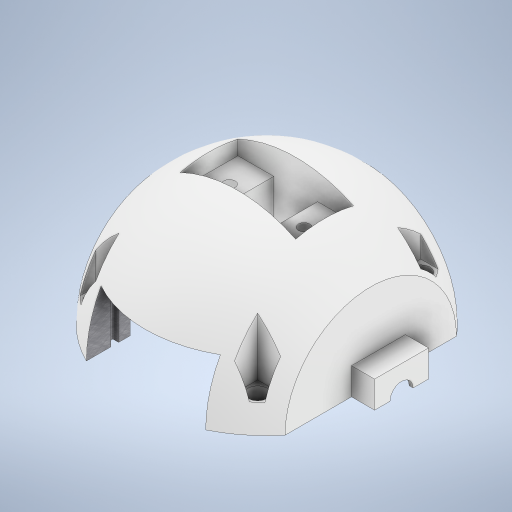
# Autodesk Inventor part: naibu-rightside
Saved by Autodesk Inventor 2023 (Build 270158000, 158)
## iProperties
Created: 2022-10-08
Part Number: naibu-rightside
Material: ABS プラスチック
Document SubType Name: Modeling
Designer: ellie
Density: 1.06 g/cm^3
Appearance: 積雪
Author: ellie
Autodesk Inventor part; units mm, degrees
ref_plane "YZ Plane" through (0, 0, 0) normal (1, 0, 0) x (0, 1, 0)
ref_plane "XZ Plane" through (0, 0, 0) normal (0, 1, 0) x (-1, 0, 0)
ref_plane "XY Plane" through (0, 0, 0) normal (0, 0, 1) x (1, 0, 0)
sketch "スケッチ1" plane through (0, 0, 0) normal (0, 1, 0) x (-1, 0, 0)
  circle A0 centre (0, 0) radius 35
  line L0 (0, 0) -> (0, -35)
  line L1 (0, 0) -> (0, 35)
  dimension "d0" = 70
  constraints: 4 end point, 2 point on circle, 2 vertical, 1 centre point, 1 coincident
  measures "d0" diameter of A0
revolve "回転1" add sketch "スケッチ1" angle 180 about axis through (0, 0, 0) along (0, 0, 1) picked at (-2.5961, -23.0408) contours L1 L0 A0
sketch "スケッチ5" plane through (0, 0, 0) normal (0, -1, 0) x (1, 0, 0)
  line L0 (-20, -23) -> (20, -23)
  line L1 (20, -23) -> (20, -13)
  line L2 (20, -13) -> (-20, -13)
  line L3 (-20, -13) -> (-20, -23)
  line L4 (-20, -15) -> (-20, -13)
  line L5 (0, 25) -> (-17, 25)
  line L6 (-17, 25) -> (-17, 23)
  line L7 (-17, 23) -> (0, 23)
  line L8 (0, 23) -> (0, 25)
  line L9 (0, 20) -> (-20, 20)
  line L10 (-20, 20) -> (-20, 19)
  line L11 (-20, 19) -> (0, 19)
  line L12 (0, 19) -> (0, 20)
  line L13 (0, 13) -> (-21, 13)
  line L14 (-21, 13) -> (-21, 11)
  line L15 (-21, 11) -> (0, 11)
  line L16 (0, 11) -> (0, 13)
  line L17 (0, 5) -> (-23, 5)
  line L18 (-23, 5) -> (-23, 3)
  line L19 (-23, 3) -> (0, 3)
  line L20 (0, 3) -> (0, 5)
  circle A0 centre (0, 0) radius 35 projected
  circle A1 centre (0, 0) radius 35 projected
  line L21 (0, 35) -> (0, -35)
  line L22 (35, 0) -> (-35, 0)
  line L23 (-32, 3) -> (-23, 3)
  line L24 (-23, 3) -> (-23, -7)
  line L25 (-23, -7) -> (-32, -7)
  line L26 (-32, -7) -> (-32, 3)
  line L27 (-23, -8.0262) -> (-23, 3)
  line L28 (-27, 22.2711) -> (-27, -22.2711)
  line L29 (-15.5, 25) -> (0, 25)
  line L30 (0, 25) -> (0, 35)
  line L31 (0, 35) -> (-15.5, 35)
  line L32 (-15.5, 35) -> (-15.5, 25)
  line L33 (-15.5, 23) -> (0, 23)
  line L34 (0, 23) -> (0, 20)
  line L35 (0, 20) -> (-15.5, 20)
  line L36 (-15.5, 20) -> (-15.5, 23)
  line L37 (-19, 13) -> (0, 13)
  line L38 (0, 13) -> (0, 19)
  line L39 (0, 19) -> (-19, 19)
  line L40 (-19, 19) -> (-19, 13)
  line L41 (-19, 11) -> (0, 11)
  line L42 (0, 11) -> (0, 5)
  line L43 (0, 5) -> (-19, 5)
  line L44 (-19, 5) -> (-19, 11)
  line L45 (-23, -2) -> (-39.6865, -2)
  line L46 (-23, -2) -> (-7.8337, -2)
  line L47 (-8, 3) -> (-23, 3)
  line L48 (-23, 3) -> (-23, -7)
  line L49 (-23, -7) -> (-8, -7)
  line L50 (-8, -7) -> (-8, 3)
  line L51 (-8, 3) -> (-23, -7) construction
  line L52 (-23, 3) -> (-8, -7) construction
  line L53 (-23, 5) -> (-33, 5)
  line L54 (-33, 5) -> (-33, -9)
  line L55 (-33, -9) -> (-23, -9)
  line L56 (-23, -9) -> (-23, 5)
  line L57 (-23, 5) -> (-33, -9) construction
  line L58 (-33, 5) -> (-23, -9) construction
  line L59 (-8, 3) -> (-1, 3)
  line L60 (-1, 3) -> (-1, -7)
  line L61 (-1, -7) -> (-8, -7)
  line L62 (-8, -7) -> (-8, 3)
  line L63 (-8, 3) -> (-1, -7) construction
  line L64 (-1, 3) -> (-8, -7) construction
  line L65 (-23, 3) -> (-27, 3)
  line L66 (-23, -7) -> (-27, -7)
  line L67 (-23, 5) -> (-27, 5)
  line L68 (-23, -9) -> (-27, -9)
  line L69 (23.4307, -26) -> (-23.4307, -26)
  line L70 (-8, 3) -> (-6.8, 3)
  line L71 (-6.8, 3) -> (-6.8, -7)
  line L72 (-6.8, -7) -> (-8, -7)
  line L73 (-8, -7) -> (-8, 3)
  line L74 (0, 5) -> (2, 5)
  line L75 (0, -3) -> (0, 5)
  line L76 (-11.5791, -13) -> (-8, -13)
  point P0 (0, -23)
  point P1 (0, -13)
  point P2 (0, 24)
  point P3 (0, 19.5)
  point P4 (0, 12)
  point P5 (0, 4)
  point P6 (-20, -18)
  point P7 (-27, -0.5262)
  point P8 (-27, -7)
  point P9 (-15.5, 21.5)
  point P10 (-15.5, 31.3807)
  point P11 (0, 25)
  point P12 (0, 23)
  point P13 (0, 11)
  point P14 (0, 13)
  point P15 (-27, 0)
  point P16 (-32, 0)
  point P17 (-23, 0)
  point P18 (-15.5, -2)
  point P19 (-28, -2)
  point P20 (-4.5, -2)
  point P21 (-8, -7)
  point P22 (-8, 3)
  point P23 (-27, 0.5)
  point P24 (-28, 0.4738)
  point P25 (-28, -11.5262)
  point P26 (-27, -11.5)
  point P27 (-23, 3)
  point P28 (-8, 0)
  point P29 (-1, 0)
  point P30 (-8, -7)
  point P31 (0, 5)
  point P32 (0, 3)
  point P33 (-27, -9)
  point P34 (-27, 5)
  dimension "d12" = 40
  dimension "d13" = 10
  dimension "d23" = 17
  dimension "d24" = 2
  dimension "d27" = 20
  dimension "d28" = 1
  dimension "d30" = 21
  dimension "d31" = 2
  dimension "d33" = 2
  dimension "d88" = 0
  dimension "d89" = 0
  dimension "d90" = 12
  dimension "d92" = 20
  dimension "d93" = 10
  dimension "d97" = 9
  dimension "d98" = 10
  dimension "d113" = 27
  dimension "d122" = 15.5
  dimension "d123" = 35
  dimension "d124" = 3
  dimension "d125" = 15.5
  dimension "d126" = 6
  dimension "d127" = 6
  dimension "d147" = 10
  dimension "d149" = 8
  dimension "d151" = 15
  dimension "d161" = 14
  dimension "d162" = 10
  dimension "d164" = 10
  dimension "d165" = 7
  dimension "d170" = 26
  dimension "d175" = 1.2
  dimension "d187" = 1
  dimension "d262" = 2
  dimension "d263" = 2
  constraints: 152 end point, 29 parallel, 19 horizontal, 17 perpendicular, 15 midpoint, 15 point on line, 9 collinear, 1 vertical, 20 other
  measures "d12" distance of L2.end L1.end
  measures "d13" distance of L1.end L0.end
  measures "d23" distance of L7.end L6.end
  measures "d24" distance of L6.end L5.end
  measures "d27" distance of L11.end L10.end
  measures "d28" distance of L10.end L9.end
  measures "d30" distance of L15.end L14.end
  measures "d31" distance of L14.end L13.end
  measures "d33" distance of L18.end L17.end
  measures "d89" distance from line of point (0, 0) L22
  measures "d90" distance from line of L0 point (0, -35)
  measures "d92" distance of the line from the sketch origin of L3
  measures "d93" distance from line of L5 point (0, 35)
  measures "d97" distance of L24.end L25.end
  measures "d98" distance of L23.end L24.end
  measures "d113" distance of the line from the sketch origin of L28
  measures "d122" distance of the line from the sketch origin of L32
  measures "d123" distance between parallel lines of L31 L22
  measures "d124" distance of L33.end L34.end
  measures "d126" distance of L38.end L37.end
  measures "d127" distance of L41.end L42.end
  measures "d147" distance of L48.end L47.end
  measures "d149" distance of the line from the sketch origin of L50
  measures "d151" distance between parallel lines of L50 L24
  measures "d161" distance between parallel lines of L55 L53
  measures "d162" distance between parallel lines of L48 L54
  measures "d164" distance between parallel lines of L61 L59
  measures "d165" distance between parallel lines of L50 L60
  measures "d170" distance between parallel lines of L69 L22
  measures "d175" distance of L71.end L72.end
  measures "d187" distance between parallel lines of L75 L60
  measures "d262" distance between parallel lines of L14 L44
  measures "d263" distance between parallel lines of L14 L40
extrude "GNSボード" cut sketch "スケッチ5" against normal blind 16 contours L8 L7 L6 L5
extrude "GNSボード止めるよう" cut sketch "スケッチ5" against normal blind 15 contours L21 L5 L32 A0 | L21 L9 L36 L7
extrude "アルミ板１" cut sketch "スケッチ5" against normal blind 20 contours L12 L11 L10 L9
extrude "メイン基板" cut sketch "スケッチ5" against normal blind 21 contours L15 L14 L13 L16
extrude "メイン止めるよう" cut sketch "スケッチ5" against normal blind 16.5 contours L17 L44 L15 L21 | L13 L40 L11 L21
extrude "アルミ板２" cut sketch "スケッチ5" against normal blind 20 contours L19 L18 L17 L20
extrude "電池ボックス入れ" cut sketch "スケッチ5" against normal blind 13 contours L3 L2 L21 L0 | L21 L2 L1 L0
extrude "side ut" cut sketch "スケッチ5" against normal blind 100 contours A0 L45 L54 L55 L28 | A0 L22 L54 L45 | L55 L54 L45 L26 L25 L28 | A0 L28 L53 L54 L22 | L54 L22 L26 L45 | L25 L26 L45 L28 | L54 L53 L28 L23 L26 L22 | L26 L22 L28 L45 | L26 L23 L28 L22
extrude "motor case" add sketch "スケッチ5" against normal blind 7 contours L55 L54 L45 L26 L25 L28 | L28 L25 L27 L56 L55 | L54 L22 L26 L45 | L28 L45 L24 L25 | L25 L26 L45 L28 | L50 L46 L24 L22 | L22 L24 L19 L50 | L54 L53 L28 L23 L26 L22 | L26 L22 L28 L45 | L24 L46 L50 L49 | L28 L22 L24 L45 | L18 L23 L28 L53 | L22 L28 L23 L24 | L26 L23 L28 L22
extrude "bottom cut" cut sketch "スケッチ5" against normal blind 90 contours L69 A0 L21 | L21 A0 L69
extrude "motor" cut sketch "スケッチ5" against normal blind 6 contours L60 L61 L71 L22 | L22 L71 L19 L60 | L71 L61 L50 L22 | L22 L50 L19 L71 | L28 L45 L24 L25 | L25 L26 L45 L28 | L50 L46 L24 L22 | L22 L24 L19 L50 | L26 L22 L28 L45 | L24 L46 L50 L49 | L28 L22 L24 L45 | L22 L28 L23 L24 | L26 L23 L28 L22
extrude "motor block" add sketch "スケッチ5" against normal blind 10 contours L71 L61 L50 L22 | L22 L50 L19 L71
sketch "スケッチ26" plane through (-33, 0, -9) normal (-1, 0, 0) x (0, 0, 1)
  line L0 (14, 0) -> (0, 0) projected
  circle A0 centre (7, 0) radius 3
  point P0 (9, 0)
  point P1 (7, 0)
  point P2 (7, 0)
  point P3 (7, 0)
  point P4 (4, 0)
  point P5 (10, 0)
  dimension "d197" = 6
  constraints: 1 centre point, 1 coincident
  measures "d197" diameter of A0
extrude "押し出し34" cut sketch "スケッチ26" against normal blind 27 contours L0 A0 picked at (7.7485, 0.6631)
mirror "ミラー11" about plane through (0, 0, 0) normal (1, 0, 0) of "GNSボード", "GNSボード止めるよう", "アルミ板１", "メイン止めるよう", "メイン基板", "アルミ板２", "motor", "押し出し34", "motor case", "電池ボックス入れ", "motor block", "side ut"
ref_plane "作業平面5" through (0, 13, 0) normal (0, -1, 0) x (1, 0, 0)
ref_plane "作業平面6" through (-15.5, 35, 25) normal (0, -1, 0) x (1, 0, 0)
sketch "スケッチ29" plane through (-15.5, 35, 25) normal (0, -1, 0) x (1, 0, 0)
  line L0 (15.5, -25) -> (-67.7134, -25)
  line L1 (-67.7134, -25) -> (15.5, -25)
  line L2 (110.7852, -24.5555) -> (110.7852, -27.3413)
  line L3 (15.5, -25) -> (98.1975, -25)
  circle A0 centre (25.2, -25) radius 1.5
  circle A1 centre (5.8, -25) radius 1.5
  line L4 (32.5, 0) -> (-1.5, 0) projected
  line L5 (15.5, 0) -> (15.5, -51)
  line L6 (-7.9307, -51) -> (38.9307, -51) projected
  dimension "d205" = 3
  dimension "d206" = 19.4
  dimension "d207" = 0
  constraints: 10 end point, 2 centre point, 2 horizontal, 2 midpoint, 1 collinear, 1 vertical, 1 other
  measures "d205" diameter of A0
  measures "d206" distance of A1.centre A0.centre
  measures "d207" distance from line of L3 A0.centre
extrude "押し出し36" cut sketch "スケッチ29" along normal blind 25
sketch "スケッチ30" plane through (-15.5, 35, 25) normal (0, -1, 0) x (1, 0, 0)
  line L0 (0.5, -17.5) -> (30.5, -17.5)
  line L1 (30.5, -17.5) -> (30.5, -32.5)
  line L2 (30.5, -32.5) -> (0.5, -32.5)
  line L3 (0.5, -32.5) -> (0.5, -17.5)
  line L4 (0.5, -17.5) -> (30.5, -32.5) construction
  line L5 (30.5, -17.5) -> (0.5, -32.5) construction
  point P0 (15.5, -25)
  dimension "d210" = 30
  dimension "d211" = 15
  constraints: 12 end point, 2 midpoint, 2 parallel, 1 horizontal, 1 perpendicular
  measures "d210" distance of L1.end L2.end
  measures "d211" distance of L0.end L1.end
extrude "押し出し37" cut sketch "スケッチ30" along normal blind 8
ref_plane "作業平面7" through (-15.5, 10, 25) normal (0, 1, 0) x (1, 0, 0)
sketch "スケッチ33" plane through (-15.5, 10, 25) normal (0, 1, 0) x (1, 0, 0)
  circle A0 centre (25.2, 25) radius 1.5 projected
  circle A1 centre (5.8, 25) radius 1.5 projected
  line L0 (0.5, 32.5) -> (0.5, 17.5) projected
  line L1 (30.5, 17.5) -> (30.5, 32.5) projected
  line L2 (0.5, 17.5) -> (30.5, 17.5) projected
  line L3 (30.5, 32.5) -> (0.5, 32.5) projected
  line L4 (15.5, 0) -> (15.5, 51) projected
  line L5 (15.5, 25) -> (98.1975, 25) projected
  circle A2 centre (25.2, 25) radius 3
  circle A3 centre (5.8, 25) radius 3
  dimension "d219" = 6
  dimension "d220" = 6
  constraints: 2 centre point, 2 coincident
  measures "d219" diameter of A2
  measures "d220" diameter of A3
extrude "押し出し39" cut sketch "スケッチ33" along normal blind 10 contours L5 A0 | L5 A2 A0 | A0 L5 A2 | A0 L5 | A1 | A3
sketch "スケッチ34" plane through (-23, 6, 3) normal (0, 0, 1) x (1, 0, 0)
  line L0 (31, 0) -> (46, 0) projected
  line L1 (46, 0) -> (46, 14) projected
  line L2 (46, 14) -> (32.7, 14) projected
  line L3 (32.7, 4) -> (32.7, 14) projected
  line L4 (32.7, 14) -> (13.3, 14) projected
  line L5 (13.3, 4) -> (13.3, 14) projected
  line L6 (13.3, 14) -> (0, 14) projected
  line L7 (0, 0) -> (0, 14) projected
  line L8 (0, 0) -> (15, 0) projected
  line L9 (15, -6) -> (15, 0) projected
  line L10 (16.2, -6) -> (15, -6) projected
  line L11 (16.2, -6) -> (16.2, 0) projected
  line L12 (16.2, 0) -> (22, 0) projected
  line L13 (22, 0) -> (22, -6) projected
  line L14 (24, -6) -> (22, -6) projected
  line L15 (24, -6) -> (24, 0) projected
  line L16 (24, 0) -> (29.8, 0) projected
  line L17 (29.8, -6) -> (29.8, 0) projected
  line L18 (29.8, -6) -> (31, -6) projected
  line L19 (31, -6) -> (31, 0) projected
  line L20 (9.8, 4) -> (16.8, 4)
  line L21 (16.8, 4) -> (16.8, 8)
  line L22 (16.8, 8) -> (9.8, 8)
  line L23 (9.8, 8) -> (9.8, 4)
  line L24 (-23.2, 4) -> (69.2, 4) projected
  line L25 (29.2, 4) -> (36.2, 4)
  line L26 (36.2, 4) -> (36.2, 8)
  line L27 (36.2, 8) -> (29.2, 8)
  line L28 (29.2, 8) -> (29.2, 4)
  point P0 (23, -6)
  point P1 (9.8, 6)
  dimension "d223" = 4
  dimension "d224" = 7
  dimension "d225" = 3.5
  dimension "d226" = 4
  dimension "d227" = 7
  dimension "d228" = 3.5
  constraints: 16 end point, 4 parallel, 2 collinear, 2 horizontal, 2 perpendicular, 1 midpoint
  measures "d223" distance between parallel lines of L20 L22
  measures "d224" distance between parallel lines of L23 L21
  measures "d225" distance from line of point (9.8, 6) L5
  measures "d226" distance of L27.end L25.start
  measures "d227" distance between parallel lines of L26 L28
  measures "d228" distance between parallel lines of L3 L28
extrude "押し出し40" cut sketch "スケッチ34" against normal blind 3 contours L24 L3 L27 L26 | L24 L28 L27 L3 | L22 L21 L20 L5 | L5 L20 L23 L22
sketch "スケッチ35" plane through (-17, 0, 23) normal (0, -1, 0) x (1, 0, 0)
  circle A0 centre (-4, 0.4) radius 2.4
  line L0 (9, -30) -> (9, -20) projected
  line L1 (-6, -20) -> (9, -20) projected
  line L2 (-15, -20) -> (-6, -20) projected
  line L3 (-15, -30) -> (-15, -20) projected
  line L4 (16, -30) -> (10.2, -30) projected
  line L5 (-16, -22) -> (-15, -22) projected
  line L6 (-15, -22) -> (-15, -20) projected
  line L7 (-15, -20) -> (-6, -20) projected
  line L8 (-6, -20) -> (-6, -18) projected
  line L9 (-6, -18) -> (-2, -18) projected
  line L10 (-2, -18) -> (-2, -12) projected
  line L11 (-2, -12) -> (-4, -12) projected
  line L12 (-4, -12) -> (-4, -10) projected
  line L13 (-4, -10) -> (-2, -10) projected
  line L14 (-2, -10) -> (-2, -4) projected
  line L15 (-2, -4) -> (-3, -4) projected
  line L16 (-3, -4) -> (-3, -3) projected
  line L17 (-3, -3) -> (1.5, -3) projected
  line L18 (1.5, -3) -> (1.5, 0) projected
  line L19 (1.5, 0) -> (0, 0) projected
  line L20 (0, 0) -> (0, 2) projected
  line L21 (0, 2) -> (1.5, 2) projected
  line L22 (1.5, 2) -> (1.5, 8.3807) projected
  arc A1 (1.5, 8.3807) -> (-10, -0.7289) centre (17, -23) ccw projected
  line L23 (-10, -0.7289) -> (-10, -18) projected
  line L24 (-10, -18) -> (-16, -18) projected
  line L25 (-16, -18) -> (-16, -22) projected
  line L26 (10.2, -20) -> (10.2, -30) projected
  line L27 (16, -20) -> (16, -30) projected
  line L28 (10.2, -20) -> (16, -20) projected
  line L29 (9, -30) -> (-15, -30) projected
  point P0 (-15, -22)
  dimension "d231" = 4.8
  dimension "d233" = 1
  dimension "d234" = 4
  constraints: 1 centre point
  measures "d231" diameter of A0
  measures "d233" distance edge to line of A0 L17
  measures "d234" distance from line of A0.centre L20
extrude "押し出し41" cut sketch "スケッチ35" against normal blind 20 contours A0
mirror "ミラー12" about plane through (0, 0, 0) normal (1, 0, 0) of "押し出し41"
sketch "スケッチ36" plane through (-33, 0, -9) normal (0, -1, 0) x (1, 0, 0)
  circle A0 centre (10, -8) radius 2.4
  line L0 (41, 4) -> (39.8, 4) projected
  line L1 (39.8, 2) -> (39.8, 4) projected
  line L2 (34, 2) -> (34, 12) projected
  line L3 (34, 12) -> (32, 12) projected
  line L4 (32, 12) -> (32, 2) projected
  line L5 (26.2, 2) -> (26.2, 4) projected
  line L6 (26.2, 4) -> (25, 4) projected
  line L7 (25, 12) -> (25, 10) projected
  line L8 (10, 12) -> (10, 14) projected
  line L9 (32, 2) -> (26.2, 2) projected
  line L10 (1, 2) -> (1, 4) projected
  line L11 (1, 4) -> (0, 4) projected
  line L12 (0, 4) -> (0, 0) projected
  line L13 (0, 0) -> (6, 0) projected
  line L14 (6, 0) -> (6, -13.2711) projected
  arc A1 (6, -13.2711) -> (9.5693, -17) centre (33, 9) ccw projected
  line L15 (9.5693, -17) -> (56.4307, -17) projected
  arc A2 (56.4307, -17) -> (60, -13.2711) centre (33, 9) ccw projected
  line L16 (60, -13.2711) -> (60, 0) projected
  line L17 (66, 0) -> (60, 0) projected
  line L18 (66, 4) -> (66, 0) projected
  line L19 (66, 4) -> (65, 4) projected
  line L20 (65, 4) -> (65, 2) projected
  line L21 (39.8, 2) -> (34, 2) projected
  line L22 (56, 14) -> (56, 12) projected
  line L23 (41, 12) -> (41, 10) projected
  line L24 (13, -4) -> (53, -4) projected
  line L25 (53, -4) -> (53, -14) projected
  line L26 (53, -14) -> (13, -14) projected
  line L27 (13, -14) -> (13, -4) projected
  line L28 (53, -4) -> (53, -14) projected
  line L29 (13, -4) -> (53, -4) projected
  line L30 (13, -14) -> (13, -4) projected
  line L31 (53, -14) -> (13, -14) projected
  line L32 (0, 10) -> (1, 10) projected
  line L33 (1, 10) -> (1, 12) projected
  line L34 (1, 12) -> (10, 12) projected
  line L35 (10, 14) -> (14, 14) projected
  line L36 (14, 14) -> (14, 20) projected
  line L37 (14, 20) -> (12, 20) projected
  line L38 (12, 20) -> (12, 22) projected
  line L39 (12, 22) -> (14, 22) projected
  line L40 (14, 22) -> (14, 28) projected
  line L41 (14, 28) -> (13, 28) projected
  line L42 (13, 28) -> (13, 29) projected
  line L43 (13, 29) -> (17.5, 29) projected
  line L44 (17.5, 29) -> (17.5, 32) projected
  line L45 (17.5, 32) -> (16, 32) projected
  line L46 (16, 32) -> (16, 34) projected
  line L47 (16, 34) -> (17.5, 34) projected
  line L48 (17.5, 34) -> (17.5, 40.3807) projected
  arc A3 (17.5, 40.3807) -> (6, 31.2711) centre (33, 9) ccw projected
  line L49 (6, 31.2711) -> (6, 14) projected
  line L50 (6, 14) -> (0, 14) projected
  line L51 (0, 14) -> (0, 10) projected
  line L52 (25, 10) -> (26.2, 10) projected
  line L53 (26.2, 10) -> (26.2, 12) projected
  line L54 (26.2, 12) -> (25, 12) projected
  line L55 (25, 4) -> (25, 2) projected
  line L56 (25, 2) -> (1, 2) projected
  line L57 (65, 2) -> (41, 2) projected
  line L58 (41, 4) -> (41, 2) projected
  line L59 (39.8, 10) -> (41, 10) projected
  line L60 (39.8, 12) -> (41, 12) projected
  line L61 (39.8, 10) -> (39.8, 12) projected
  line L62 (65, 10) -> (66, 10) projected
  line L63 (66, 14) -> (66, 10) projected
  line L64 (60, 14) -> (66, 14) projected
  line L65 (60, 14) -> (60, 31.2711) projected
  arc A4 (60, 31.2711) -> (48.5, 40.3807) centre (33, 9) ccw projected
  line L66 (48.5, 40.3807) -> (48.5, 34) projected
  line L67 (48.5, 34) -> (50, 34) projected
  line L68 (50, 34) -> (50, 32) projected
  line L69 (50, 32) -> (48.5, 32) projected
  line L70 (48.5, 32) -> (48.5, 29) projected
  line L71 (48.5, 29) -> (53, 29) projected
  line L72 (53, 29) -> (53, 28) projected
  line L73 (53, 28) -> (52, 28) projected
  line L74 (52, 28) -> (52, 22) projected
  line L75 (52, 22) -> (54, 22) projected
  line L76 (54, 22) -> (54, 20) projected
  line L77 (54, 20) -> (52, 20) projected
  line L78 (52, 20) -> (52, 14) projected
  line L79 (52, 14) -> (56, 14) projected
  line L80 (56, 12) -> (65, 12) projected
  line L81 (65, 12) -> (65, 10) projected
  circle A5 centre (12, 32.4) radius 2.4 projected
  circle A6 centre (54, 32.4) radius 2.4 projected
  dimension "d237" = 4.8
  dimension "d238" = 3
  dimension "d239" = 10
  constraints: 1 centre point
  measures "d237" diameter of A0
  measures "d238" distance from line of A0.centre L27
  measures "d239" distance from line of A0.centre L9
extrude "押し出し42" cut sketch "スケッチ36" against normal blind 25 contours A0
mirror "ミラー13" about plane through (0, 0, 0) normal (1, 0, 0) of "押し出し42"
ref_plane "作業平面8" through (-17, 35, 23) normal (0, -1, 0) x (1, 0, 0)
sketch "スケッチ37" plane through (-17, 35, 23) normal (0, -1, 0) x (1, 0, 0)
  line L0 (38, -10) -> (-4, -10) projected
  line L1 (2, -15.5) -> (2, -30.5) projected
  line L2 (2, -30.5) -> (32, -30.5) projected
  line L3 (32, -30.5) -> (32, -15.5) projected
  line L4 (32, -15.5) -> (2, -15.5) projected
  arc A0 (32.5, 4.5636) -> (1.5, 4.5636) centre (17, -23) ccw projected
  line L5 (32.5, 4.5636) -> (32.5, 8.3807) projected
  arc A1 (44, -0.7289) -> (32.5, 8.3807) centre (17, -23) ccw projected
  line L6 (44, -0.7289) -> (44, -45.2711) projected
  arc A2 (40.4307, -49) -> (44, -45.2711) centre (17, -23) ccw projected
  line L7 (40.4307, -49) -> (-6.4307, -49) projected
  arc A3 (-10, -45.2711) -> (-6.4307, -49) centre (17, -23) ccw projected
  line L8 (-10, -45.2711) -> (-10, -0.7289) projected
  arc A4 (1.5, 8.3807) -> (-10, -0.7289) centre (17, -23) ccw projected
  line L9 (1.5, 8.3807) -> (1.5, 4.5636) projected
  line L10 (-7, 3.4) -> (-1, 3.4)
  line L11 (-1, 3.4) -> (-1, -2.6)
  line L12 (-1, -2.6) -> (-7, -2.6)
  line L13 (-7, -2.6) -> (-7, 3.4)
  arc A5 (37.6, -40) -> (37.6, -40) centre (-4, 0.4) ccw projected
  line L14 (-7, 3.4) -> (-1, -2.6) construction
  line L15 (-1, 3.4) -> (-7, -2.6) construction
  line L16 (41, 3.4) -> (35, 3.4)
  line L17 (35, 3.4) -> (35, -2.6)
  line L18 (35, -2.6) -> (41, -2.6)
  line L19 (41, -2.6) -> (41, 3.4)
  arc A6 (37.6, -40) -> (37.6, -40) centre (38, 0.4) ccw projected
  line L20 (41, 3.4) -> (35, -2.6) construction
  line L21 (35, 3.4) -> (41, -2.6) construction
  line L22 (-3, -37) -> (-9, -37)
  line L23 (-9, -37) -> (-9, -43)
  line L24 (-9, -43) -> (-3, -43)
  line L25 (-3, -43) -> (-3, -37)
  circle A7 centre (-6, -40) radius 2.4 projected
  line L26 (-3, -37) -> (-9, -43) construction
  line L27 (-9, -37) -> (-3, -43) construction
  line L28 (43, -37) -> (37, -37)
  line L29 (37, -37) -> (37, -43)
  line L30 (37, -43) -> (43, -43)
  line L31 (43, -43) -> (43, -37)
  circle A8 centre (40, -40) radius 2.4 projected
  line L32 (43, -37) -> (37, -43) construction
  line L33 (37, -37) -> (43, -43) construction
  point P0 (36.5, 1.5)
  point P1 (-2.5, 1.5)
  dimension "d243" = 6
  dimension "d244" = 6
  dimension "d245" = 6
  dimension "d246" = 6
  dimension "d247" = 6
  dimension "d248" = 6
  dimension "d249" = 6
  dimension "d250" = 6
  constraints: 48 end point, 8 midpoint, 8 parallel, 4 horizontal, 4 perpendicular, 8 other
  measures "d243" distance of L11.end L12.end
  measures "d244" distance of L10.end L11.end
  measures "d245" distance of L18.end L17.end
  measures "d246" distance of L17.end L16.end
  measures "d247" distance of L24.end L23.end
  measures "d248" distance of L23.end L22.end
  measures "d249" distance of L30.end L29.end
  measures "d250" distance of L29.end L28.end
extrude "押し出し43" cut sketch "スケッチ37" along normal blind 20 contours L29 L28 A5 A8 A6 | A6 A5 L29 | A8 A6 L31 L30 L29 A5 | A8 A5 | A5 A8 A6 | A6 A8 | A5 L28 L31 A6 A8 | L25 L24 L23 L22 | A7
extrude "押し出し44" cut sketch "スケッチ37" along normal blind 28 contours A6 L10 L11 L12 | L12 L13 A4 L10 A6 | L13 L10 A4 | L19 L18 L17 L16 A1 | A1 L16 L19
sketch "スケッチ39" plane through (-15.5, 27, 25) normal (0, 1, 0) x (1, 0, 0)
  line L0 (21.2, 17.5) -> (9.8, 17.5)
  line L1 (9.8, 17.5) -> (9.8, 32.5)
  line L2 (9.8, 32.5) -> (21.2, 32.5)
  line L3 (21.2, 32.5) -> (21.2, 17.5)
  line L4 (21.2, 17.5) -> (9.8, 32.5) construction
  line L5 (9.8, 17.5) -> (21.2, 32.5) construction
  circle A0 centre (5.8, 25) radius 1.5 projected
  circle A1 centre (25.2, 25) radius 1.5 projected
  line L6 (0.5, 17.5) -> (30.5, 17.5) projected
  line L7 (30.5, 32.5) -> (0.5, 32.5) projected
  circle A2 centre (5.8, 25) radius 1.5 projected
  circle A3 centre (25.2, 25) radius 1.5 projected
  line L8 (0.5, 32.5) -> (30.5, 32.5) projected
  line L9 (0.5, 17.5) -> (0.5, 32.5) projected
  line L10 (30.5, 17.5) -> (0.5, 17.5) projected
  line L11 (30.5, 32.5) -> (30.5, 17.5) projected
  point P0 (15.5, 25)
  dimension "d255" = 4
  dimension "d256" = 0
  constraints: 12 end point, 2 midpoint, 2 parallel, 1 horizontal, 1 perpendicular
  measures "d255" distance from line of L1 A0.centre
  measures "d256" distance between parallel lines of L6 L0
extrude "押し出し45" cut sketch "スケッチ39" against normal up to surface (10.5 mm away) contours L0 L1 L2 L3
sketch "スケッチ40" plane through (0, 16.5, 0) normal (0, -1, 0) x (1, 0, 0)
  line L0 (-5.7, 7.5) -> (5.7, 7.5)
  line L1 (5.7, 7.5) -> (5.7, 11)
  line L2 (5.7, 11) -> (-5.7, 11)
  line L3 (-5.7, 11) -> (-5.7, 7.5)
  line L4 (-5.7, 7.5) -> (5.7, 7.5) projected
  line L5 (5.7, 7.5) -> (5.7, 5) projected
  line L6 (-5.7, 5) -> (-5.7, 7.5) projected
  line L7 (-5.7, 7.5) -> (-15, 7.5) projected
  line L8 (-5.7, 5) -> (-5.7, 7.5) projected
  line L9 (-5.7, 7.5) -> (5.7, 7.5) projected
  line L10 (5.7, 7.5) -> (5.7, 5) projected
  line L11 (19, 5) -> (5.7, 5) projected
  line L12 (19, 5) -> (19, 11) projected
  line L13 (-19, 11) -> (19, 11) projected
  line L14 (-19, 5) -> (-19, 11) projected
  line L15 (-5.7, 5) -> (-19, 5) projected
  line L16 (-5.7, 3) -> (-5.7, 5) projected
  line L17 (-5.7, 5) -> (-23, 5) projected
  line L18 (-23, 3) -> (-23, 5) projected
  line L19 (-9.7, 3) -> (-23, 3) projected
  line L20 (-5.7, 3) -> (-9.7, 3) projected
  line L21 (5.7, 5) -> (5.7, 3) projected
  line L22 (9.7, 3) -> (5.7, 3) projected
  line L23 (23, 3) -> (9.7, 3) projected
  line L24 (23, 3) -> (23, 5) projected
  line L25 (23, 5) -> (5.7, 5) projected
  line L26 (21, 11) -> (-21, 11) projected
  line L27 (21, 11) -> (21, 13) projected
  line L28 (21, 13) -> (-21, 13) projected
  line L29 (-21, 11) -> (-21, 13) projected
  line L30 (-5.7, 3) -> (-5.7, 5) projected
  line L31 (-5.7, 5) -> (-23, 5) projected
  line L32 (-23, 3) -> (-23, 5) projected
  line L33 (-9.7, 3) -> (-23, 3) projected
  line L34 (-5.7, 3) -> (-9.7, 3) projected
  line L35 (5.7, 5) -> (5.7, 3) projected
  line L36 (9.7, 3) -> (5.7, 3) projected
  line L37 (23, 3) -> (9.7, 3) projected
  line L38 (23, 3) -> (23, 5) projected
  line L39 (23, 5) -> (5.7, 5) projected
  point P0 (0, 0)
  dimension "d259" = 3.5
  constraints: 8 end point, 3 collinear, 2 parallel, 1 horizontal, 1 perpendicular
  measures "d259" distance between parallel lines of L2 L0
extrude "押し出し46" cut sketch "スケッチ40" against normal blind 10 contours L3 L2 L1 L0
